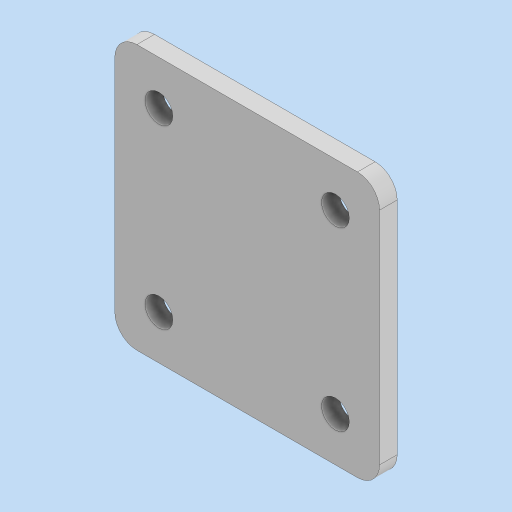
# Autodesk Inventor part: Base Profile-Connector-Plate
Saved by Autodesk Inventor 2023.2 (Build 272271000, 271)
## iProperties
Created: 2024-02-21
Part Number: Base Profile-Connector-Plate
Material: Generisch
Document SubType Name: Modeling
Designer: Nils Bade
Density: 1 g/cm^3
Appearance: Vorgabe
Description: Fertigung
Auf Bestellliste: True
Author: Nils Bade
Autodesk Inventor part; units mm, degrees
ref_plane "YZ Plane" through (0, 0, 0) normal (1, 0, 0) x (0, 1, 0)
sketch "S-BasePlate" plane through (0, 0, 0) normal (0, 0, 1) x (1, 0, 0)
  line L0 (-30, 30) -> (30, 30)
  line L1 (30, 30) -> (30, -30)
  line L2 (30, -30) -> (-30, -30)
  line L3 (-30, -30) -> (-30, 30)
  line L4 (-30, 30) -> (30, -30) construction
  line L5 (30, 30) -> (-30, -30) construction
  line L6 (-30, 20) -> (30, 20) construction
  line L7 (-42, 0) -> (42, 0) construction
  circle A0 centre (-20, 20) radius 3.15
  line L8 (0, 42) -> (0, -42) construction
  circle A1 centre (20, 20) radius 3.15
  circle A2 centre (-20, -20) radius 3.15
  circle A3 centre (20, -20) radius 3.15
  point P0 (0, 0)
  dimension "d0" = 60
  dimension "d1" = 60
  dimension "d2" = 20
  dimension "d3" = 6.3
  constraints: 14 end point, 4 centre point, 4 point on line, 3 symmetric about line, 2 midpoint, 2 parallel, 2 perpendicular, 1 horizontal, 3 other
  measures "d0" distance of L1.end L2.end
  measures "d1" distance of L2.end L0.start
  measures "d2" distance between parallel lines of L7 L6
  measures "d3" diameter of A0
extrude "Ex-BasePlate" add sketch "S-BasePlate" along normal blind 4
fillet "Rundung-2mm" radius 5 4 edges at (-30, -30, 2) (-30, 30, 2) (30, 30, 2) (30, -30, 2)
ref_plane "Hilfsebene-Pos1" through (-30, 20, 0) normal (0, 1, 0) x (1, 0, 0)
ref_plane "Hilfsebene-Pos2" through (20, -20, 0) normal (0, 1, 0) x (-1, 0, 0)
